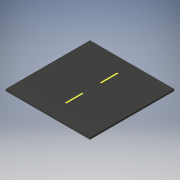
# Autodesk Inventor part: road_empty
Saved by Autodesk Inventor 2019 (Build 230136000, 136)
## iProperties
Created: 2020-04-29
Part Number: road_empty
Material: Generic
Document SubType Name: Modeling
Designer: infinity
Density: 1 g/cm^3
Appearance: Smooth - Black
Author: infinity
Autodesk Inventor part; units mm, degrees
ref_plane "YZ Plane" through (0, 0, 0) normal (1, 0, 0) x (0, 1, 0)
ref_plane "XZ Plane" through (0, 0, 0) normal (0, 1, 0) x (-1, 0, 0)
ref_plane "XY Plane" through (0, 0, 0) normal (0, 0, 1) x (1, 0, 0)
sketch "Sketch1" plane through (0, 0, 0) normal (0, 1, 0) x (-1, 0, 0)
  line L0 (0, 0) -> (1219.2, 0)
  line L1 (1219.2, 0) -> (1219.2, -1219.2)
  line L2 (1219.2, -1219.2) -> (0, -1219.2)
  line L3 (0, -1219.2) -> (0, 0)
  dimension "d0" = 1219.2
  dimension "d1" = 1219.2
  constraints: 8 end point, 2 parallel, 1 horizontal, 1 perpendicular
  measures "d0" distance of L0.end L1.end
  measures "d1" distance of L1.end L2.end
extrude "Extrusion1" add sketch "Sketch1" along normal blind 25.4
sketch "Sketch2" plane through (0, 25.4, 0) normal (0, 1, 0) x (1, 0, 0)
  line L0 (-609.6, -1656.7277) -> (-609.6, 2305.4787) construction
  line L1 (-1219.2, 1219.2) -> (-1219.2, 0) projected
  line L2 (-621.8103, 254) -> (-596.4103, 254)
  line L3 (-596.4103, 254) -> (-596.4103, 508)
  line L4 (-596.4103, 508) -> (-621.8103, 508)
  line L5 (-621.8103, 508) -> (-621.8103, 254)
  line L6 (-1219.2, 0) -> (0, 0) projected
  line L7 (-621.8103, 762) -> (-596.4103, 762)
  line L8 (-596.4103, 762) -> (-596.4103, 1016)
  line L9 (-596.4103, 1016) -> (-621.8103, 1016)
  line L10 (-621.8103, 1016) -> (-621.8103, 762)
  dimension "d4" = 609.6
  dimension "d5" = 25.4
  dimension "d6" = 254
  dimension "d7" = 254
  dimension "d10" = 508
  constraints: 18 end point, 2 parallel, 2 vertical, 1 collinear, 1 horizontal, 1 perpendicular, 7 other
  measures "d4" distance between parallel lines of L0 L1
  measures "d5" distance between parallel lines of L3 L5
  measures "d6" distance between parallel lines of L4 L2
  measures "d7" distance between parallel lines of L6 L2
  measures "d10" distance of L2.start L7.start
extrude "Extrusion2" add sketch "Sketch2" along normal blind 0.254
body "Solid1"
